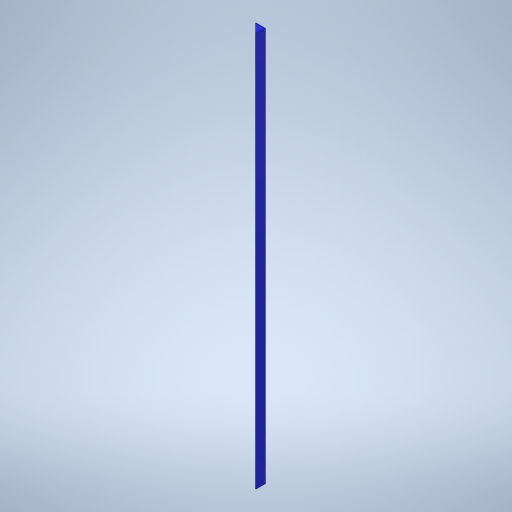
# Autodesk Inventor part: 3 x 3.25 steel side slit for 5x10
Saved by Autodesk Inventor 2024.2 (Build 282272000, 272)
## iProperties
Created: 2017-12-18
Part Number: 3 x 3.25 steel side slit for 5x10
Material: Steel
Document SubType Name: Modeling
Designer: torba
Density: 7.85 g/cm^3
Appearance: Blue - Wall Paint - Glossy
Author: torba
Autodesk Inventor part; units mm, degrees
ref_plane "YZ Plane" through (0, 0, 0) normal (1, 0, 0) x (0, 1, 0)
ref_plane "XZ Plane" through (0, 0, 0) normal (0, 1, 0) x (-1, 0, 0)
ref_plane "XY Plane" through (0, 0, 0) normal (0, 0, 1) x (1, 0, 0)
sketch "Sketch1" plane through (0, 0, 0) normal (0, 1, 0) x (-1, 0, 0)
  line L0 (0, 0) -> (0, -76.2)
  line L1 (0, -76.2) -> (76.2, -76.2)
  line L2 (76.2, -76.2) -> (76.2, -69.85)
  line L3 (76.2, -69.85) -> (6.35, -69.85)
  line L4 (6.35, -69.85) -> (6.35, 0)
  line L5 (6.35, 0) -> (0, 0)
  dimension "d0" = 76.2
  dimension "d1" = 76.2
  dimension "d2" = 6.35
  dimension "d3" = 6.35
  constraints: 12 end point, 5 perpendicular, 1 vertical
  measures "d0" distance of L0.start L0.end
  measures "d1" distance of L0.end L1.end
  measures "d2" distance between parallel lines of L1 L3
  measures "d3" distance between parallel lines of L0 L4
extrude "Extrusion1" add sketch "Sketch1" along normal blind 3187.7
fillet "Fillet1" radius 3.175 2 edges at (-6.35, 1593.85, 0) (-76.2, 1593.85, -69.85)
sketch "Sketch5" plane through (0, 0, -76.2) normal (0, 0, -1) x (-1, 0, 0)
  line L0 (76.2, 0) -> (76.2, 3187.7) projected
  line L1 (76.2, 76.2) -> (38.1, 76.2)
  line L2 (38.1, 76.2) -> (38.1, 80.9625)
  line L3 (38.1, 80.9625) -> (76.2, 80.9625)
  line L4 (76.2, 80.9625) -> (76.2, 76.2)
  line L5 (0, 0) -> (76.2, 0) projected
  dimension "d39" = 38.1
  dimension "d40" = 4.7625
  dimension "d41" = 76.2
  constraints: 8 end point, 2 parallel, 1 horizontal, 1 perpendicular, 1 point on line
  measures "d39" distance of L2.end L3.end
  measures "d40" distance of L1.end L2.end
  measures "d41" distance between parallel lines of L5 L1
extrude "Extrusion5" cut sketch "Sketch5" against normal blind 254
pattern_linear "Rectangular Pattern2" count 17 spacing 75.1078 along (0, 1, 0) of "Extrusion5"
body "Solid1"
